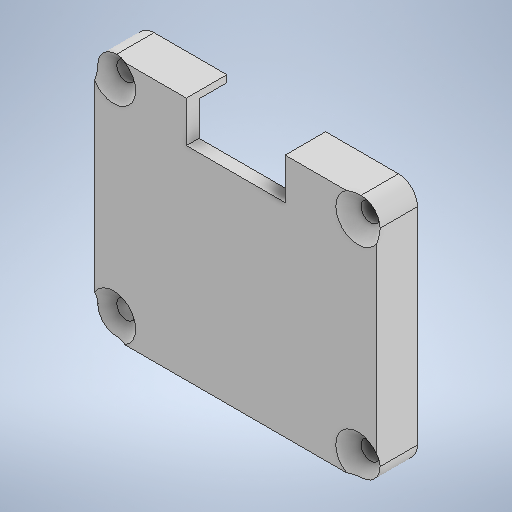
# Autodesk Inventor part: akkum_cap_pd
Saved by Autodesk Inventor 2025 (Build 290162000, 162)
## iProperties
Created: 2026-06-28
Part Number: akkum_cap_pd
Material: Типовые
Document SubType Name: Modeling
Designer: garin
Density: 1 g/cm^3
Appearance: По умолчанию
Author: garin
Autodesk Inventor part; units mm, degrees
ref_plane "YZ Plane" through (0, 0, 0) normal (1, 0, 0) x (0, 1, 0)
ref_plane "XZ Plane" through (0, 0, 0) normal (0, 1, 0) x (-1, 0, 0)
ref_plane "XY Plane" through (0, 0, 0) normal (0, 0, 1) x (1, 0, 0)
sketch "Эскиз1" plane through (0, 0, 0) normal (0, 0, 1) x (1, 0, 0)
  arc A0 (-22.3, -16.3) -> (-19.3, -19.3) centre (-19.3, -16.3) ccw
  line L0 (-22.3, -16.3) -> (-22.3, 16.3)
  arc A1 (-19.3, 19.3) -> (-22.3, 16.3) centre (-19.3, 16.3) ccw
  line L1 (-19.3, 19.3) -> (19.3, 19.3)
  arc A2 (22.3, 16.3) -> (19.3, 19.3) centre (19.3, 16.3) ccw
  line L2 (22.3, 16.3) -> (22.3, -16.3)
  arc A3 (19.3, -19.3) -> (22.3, -16.3) centre (19.3, -16.3) ccw
  line L3 (19.3, -19.3) -> (-19.3, -19.3)
  circle A4 centre (19.3, 16.3) radius 2 construction
  circle A5 centre (-19.3, 16.3) radius 2 construction
  circle A6 centre (-19.3, -16.3) radius 2 construction
  circle A7 centre (19.3, -16.3) radius 2 construction
  arc A8 (-1.4869, 14.15) -> (-14.15, 1.4869) centre (-9.15, 9.15) ccw
  line L4 (-14.15, 1.4869) -> (-14.15, -1.4869)
  arc A9 (-14.15, -1.4869) -> (-1.4869, -14.15) centre (-9.15, -9.15) ccw
  line L5 (-1.4869, -14.15) -> (1.4869, -14.15)
  arc A10 (1.4869, -14.15) -> (14.15, -1.4869) centre (9.15, -9.15) ccw
  line L6 (14.15, -1.4869) -> (14.15, 1.4869)
  arc A11 (14.15, 1.4869) -> (1.4869, 14.15) centre (9.15, 9.15) ccw
  line L7 (1.4869, 14.15) -> (-1.4869, 14.15)
  line L8 (-9.15, 9.15) -> (-9.15, 18.3) construction
  line L9 (9.15, 9.15) -> (9.15, 18.3) construction
  line L10 (-9.15, 9.15) -> (-18.3, 9.15) construction
  line L11 (-9.15, -9.15) -> (-18.3, -9.15) construction
  line L12 (-18.3, 9.15) -> (-18.3, -9.15)
  line L13 (-9.15, 18.3) -> (9.15, 18.3)
  line L14 (-22.3, 0) -> (22.3, 0) construction
  line L15 (0, 19.3) -> (0, -19.3) construction
  line L16 (18.3, 9.15) -> (18.3, -9.15)
  line L17 (-9.15, -18.3) -> (9.15, -18.3)
  circle A12 centre (-19.3, 16.3) radius 1.5
  circle A13 centre (19.3, 16.3) radius 1.5
  circle A14 centre (19.3, -16.3) radius 1.5
  circle A15 centre (-19.3, -16.3) radius 1.5
  line L18 (0, 19.3) -> (-7.8, 19.3) construction
  line L19 (-7.8, 19.3) -> (-7.8, 12.8) construction
  line L20 (-7.8, 12.8) -> (0, 12.8) construction
  line L21 (0, 12.8) -> (0, 19.3) construction
  line L22 (-7.8, 12.8) -> (7.8, 12.8)
  line L23 (7.8, 12.8) -> (7.8, 19.3)
  line L24 (7.8, 19.3) -> (-7.8, 19.3)
  line L25 (-7.8, 19.3) -> (-7.8, 12.8)
  line L26 (-18.3, 9.15) -> (-18.3, 4.15) construction
  line L27 (-18.3, -9.15) -> (-18.3, -4.15) construction
  line L28 (-18.3, -4.15) -> (-21.5, -4.15)
  line L29 (-21.5, -4.15) -> (-21.5, 4.15)
  line L30 (-21.5, 4.15) -> (-18.3, 4.15)
  line L31 (-18.3, 4.15) -> (-18.3, -4.15)
  line L32 (18.3, -4.15) -> (21.5, -4.15)
  line L33 (21.5, -4.15) -> (21.5, 4.15)
  line L34 (21.5, 4.15) -> (18.3, 4.15)
  line L35 (18.3, 4.15) -> (18.3, -4.15)
  line L36 (-21.5, 0) -> (-21.5, 12.8)
  line L37 (-21.5, 12.8) -> (-17.5405, 12.8)
  line L38 (-21.5, 0) -> (-21.5, -12.8)
  line L39 (-21.5, -12.8) -> (-17.5405, -12.8)
  point P0 (7.8, 18.1999)
  point P1 (-7.8, 18.1999)
  dimension "d5" = 3
  dimension "d6" = 3
  dimension "d7" = 3
  dimension "d8" = 3
  dimension "d9" = 7.8
  dimension "d10" = 6.5
  dimension "d11" = 15.6
  dimension "d12" = 6.5
  dimension "d13" = 5
  dimension "d14" = 5
  dimension "d15" = 3.2
  dimension "d16" = 8.3
  dimension "d19" = 12.8
  constraints: 80 end point, 22 point on circle, 16 centre point, 10 symmetric about line, 8 horizontal, 8 parallel, 6 perpendicular, 6 vertical, 5 midpoint, 4 coincident, 3 tangent, 2 point on line, 40 other
  measures "d5" diameter of A12
  measures "d6" diameter of A13
  measures "d7" diameter of A14
  measures "d8" diameter of A15
  measures "d9" distance of L20.end L19.end
  measures "d10" distance of L19.end L18.end
  measures "d11" distance of L24.end L23.end
  measures "d12" distance of L23.end L22.end
  measures "d13" distance of L10.end L26.end
  measures "d14" distance of L11.end L27.end
  measures "d15" distance of L29.end L30.end
  measures "d16" distance of L28.end L29.end
  measures "d19" distance of L36.start L36.end
extrude "Выдавливание1" add sketch "Эскиз1" along normal blind 6.4 contours L0 A1 L1 L25 L13 A8 L37 L36 L29 L38 L39 A9 L17 A10 L16 L32 L33 L34 A11 L23 A2 L2 A3 L3 A0 | L25 A8 L13 | L13 A11 L23 | A8 L25 L22 L23 A11 L6 A10 L5 A9 L4 | A8 L12 L30 L36 L37 | L16 A10 L6 A11 | A8 L4 A9 L12 | L34 L33 L32 L16 | L12 L28 L29 L30 | L12 A9 L39 L38 L28 | L17 A9 L5 A10
chamfer "Фаска1" distance 2 angle 45 4 edges at (17.8, 16.3, 6.4) (-20.8, 16.3, 6.4) (-20.8, -16.3, 6.4) (17.8, -16.3, 6.4)
extrude "Выдавливание2" cut sketch "Эскиз1" along normal blind 4.4 contours A8 L25 L22 L23 A11 L6 A10 L5 A9 L4 | A8 L12 L30 L36 L37 | L16 A10 L6 A11 | A8 L4 A9 L12 | L34 L33 L32 L16 | L12 L28 L29 L30 | L12 A9 L39 L38 L28 | L17 A9 L5 A10
sketch "Эскиз2" plane through (-22.3, -16.3, 0) normal (-1, 0, 0) x (0, 0, 1)
  line L0 (0, -3) -> (0, 0) projected
  line L1 (0, 35.6) -> (5.9, 35.6) projected
  line L2 (0, -3) -> (0, 35.6) construction
  line L3 (0, 16.3) -> (6.4, 16.3) construction
  line L4 (6.4, 30.7972) -> (6.4, 1.8028) projected
  line L5 (0, 16.3) -> (1, 16.3) construction
  line L6 (1, 16.3) -> (1, 20.5) construction
  line L7 (1, 20.5) -> (0, 20.5) construction
  line L8 (0, 20.5) -> (0, 16.3) construction
  line L9 (1, 20.5) -> (3.6, 20.5)
  line L10 (3.6, 20.5) -> (3.6, 12.1)
  line L11 (3.6, 12.1) -> (1, 12.1)
  line L12 (1, 12.1) -> (1, 20.5)
  line L13 (1, 20.5) -> (2.3, 20.5) construction
  line L14 (2.3, 20.5) -> (2.3, 19.2) construction
  line L15 (2.3, 19.2) -> (1, 19.2) construction
  line L16 (1, 19.2) -> (1, 20.5) construction
  arc A0 (3.6, 19.2) -> (1, 19.2) centre (2.3, 19.2) ccw
  arc A1 (1, 13.4) -> (3.6, 13.4) centre (2.3, 13.4) ccw
  point P0 (3.6, 13.4)
  point P1 (1, 19.2)
  point P2 (1, 13.4)
  point P3 (2.3, 12.1)
  point P4 (2.3, 20.5)
  dimension "d20" = 1
  dimension "d21" = 4.2
  dimension "d22" = 2.6
  dimension "d23" = 8.4
  dimension "d24" = 1.3
  dimension "d25" = 1.3
  constraints: 28 end point, 6 parallel, 5 point on circle, 3 horizontal, 3 perpendicular, 3 symmetric about line, 2 centre point, 2 point on line, 1 midpoint, 1 vertical, 1 other
  measures "d20" distance of L7.end L6.end
  measures "d21" distance of L6.end L5.end
  measures "d22" distance of L10.end L11.end
  measures "d23" distance of L9.end L10.end
  measures "d24" distance of L14.end L15.end
  measures "d25" distance of L13.end L14.end
extrude "Выдавливание3" cut sketch "Эскиз2" against normal blind 0.8 contours A0 L10 A1 L12
